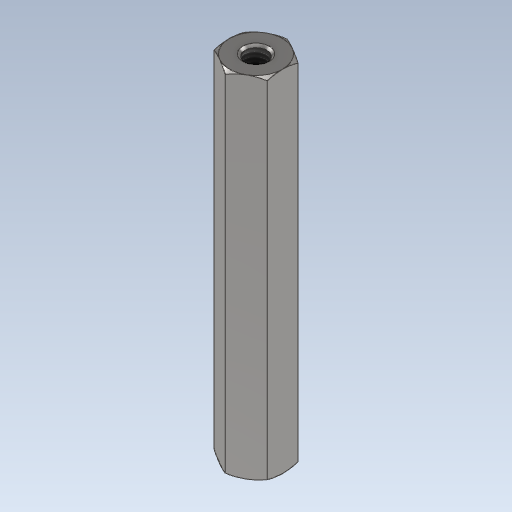
# Autodesk Inventor part: SLSBF6-39.5-M3-N3
Saved by Autodesk Inventor 2020.4 (Build 244396000, 396)
## iProperties
Part Number: SLSBF6-39.5-M3-N3
Material: ステンレス鋼 AISI 304
Document SubType Name: Modeling
Designer: Masato Kubotera
Density: 6.14131 g/cm^3
Appearance: 半つや出し
Catalog Web Link: https://jp.misumi-ec.com/vona2/detail/110300206620/?HissuCode=SLSBF6-39.5-M3-N3
Description: ReadyMade
Mass: 7.192 g
Surface Area: 9.7245 cm^2
Volume: 1.17108 cm^3
Author: Masato Kubotera
Autodesk Inventor part; units mm, degrees
ref_plane "YZ Plane" through (0, 0, 0) normal (1, 0, 0) x (0, 1, 0)
ref_plane "XZ Plane" through (0, 0, 0) normal (0, 1, 0) x (-1, 0, 0)
ref_plane "XY Plane" through (0, 0, 0) normal (0, 0, 1) x (1, 0, 0)
sketch "スケッチ1" plane through (0, 0, 0) normal (1, 0, 0) x (0, 1, 0)
  line L0 (-19.75, 0) -> (19.75, 0)
  line L1 (0, 0) -> (0, 3.4641) construction
  line L2 (-19.4821, 3.4641) -> (-19.75, 3)
  line L3 (-19.75, 3) -> (-19.75, 0)
  line L4 (-19.4821, 3.4641) -> (19.4821, 3.4641)
  line L5 (19.4821, 3.4641) -> (19.75, 3)
  line L6 (19.75, 3) -> (19.75, 0)
  dimension "d1" = 3
  dimension "d2" = 3.4641
  dimension "d3" = 30
  dimension "d4" = 39.5
  constraints: 14 end point, 3 perpendicular, 2 midpoint, 1 coincident, 1 horizontal, 1 symmetric about line
  measures "d1" distance of L0.start L2.end
  measures "d2" vertical distance of L0.start L2.start
  measures "d3" angle of L3 L2
  measures "d4" distance of L0.start L0.end
revolve "回転1" add sketch "スケッチ1" angle 360 about axis through (0, -19.75, 0) along (0, 1, 0)
sketch "スケッチ2" plane through (0, 19.75, 0) normal (0, 1, 0) x (1, 0, 0)
  circle A0 centre (0, 0) radius 3.4641 projected
  line L0 (0, -3.4641) -> (-3, -1.7321)
  line L1 (-3, -1.7321) -> (-3, 1.7321)
  line L2 (-3, 1.7321) -> (0, 3.4641)
  line L3 (0, 3.4641) -> (3, 1.7321)
  line L4 (3, 1.7321) -> (3, -1.7321)
  line L5 (3, -1.7321) -> (0, -3.4641)
  point P0 (0, 0)
  point P1 (0, 0)
  point P2 (3, -1.7321)
  point P3 (3, -1.7321)
  point P4 (3, 1.7321)
  point P5 (3, 1.7321)
  point P6 (0, 3.4641)
  point P7 (0, 3.4641)
  point P8 (-3, 1.7321)
  point P9 (-3, 1.7321)
  point P10 (-3, -1.7321)
  point P11 (-3, -1.7321)
  constraints: 12 end point, 2 coincident, 1 vertical, 15 other
extrude "押し出し1" cut sketch "スケッチ2" against normal through all contours A0 L4 | L3 A0 | A0 L5 | L2 A0 | A0 L0 | L1 A0
hole "穴1" at (0, 19.75, 0) direction (0, -1, 0) diameter 2.459 depth 6 tip angle 118 countersink diameter 3 countersink angle 90 thread size "M3x0.5" class "6H" standard "ISO Metric profile"
mirror "ミラー1" about plane through (0, 0, 0) normal (0, 1, 0) of "穴1"
equation "\"d2\" = 1.1547 * d1"
